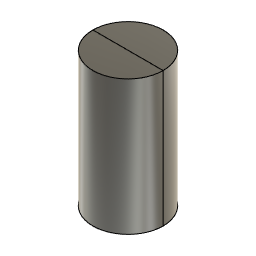
Vertical Split Can Base (Autodesk Fusion 360 design; units mm, degrees)
Autodesk Fusion 360 part; units mm, degrees
sketch "Profile" plane through (0, 0, 0) normal (1, 0, 0) x (0, 1, 0)
  line L0 (0, 0) -> (30, 0)
  line L1 (30, 0) -> (30, 115)
  line L2 (30, 115) -> (0, 115)
  line L3 (0, 2) -> (28, 2)
  line L4 (28, 2) -> (28, 113)
  line L5 (28, 113) -> (0, 113)
  line L6 (0, 115) -> (0, 113)
  line L7 (0, 2) -> (0, 0)
  dimension "d1" = 30
  dimension "d2" = 115
  dimension "d4" = -2
  constraint coincident L0.start L7.end
  constraint horizontal L0
  constraint perpendicular L0 L1
  constraint perpendicular L1 L2
  constraint perpendicular L0 L7
  measures "d1" distance of L0.start L0.end
  measures "d2" distance of L0.end L1.end
revolve "Revolve1" add sketch "Profile" angle 360 about axis through (0, 0, 1.75) along (0, 0, 1) makes body 1
split "Split1" by plane through (0, 0, 0) normal (0, 1, 0) bodies 1 makes body 2 at (-17.4017, 24.4373, 38.3333)
named bodies: "Front Half", "Back Half"
